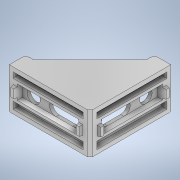
# Autodesk Inventor part: 3030 corner bracket 60x30
Saved by Autodesk Inventor 2022 (Build 260153000, 153)
## iProperties
Created: 2022-09-17
Part Number: 3030 corner bracket 60x30
Material: Genérico
Document SubType Name: Modeling
Designer: JK
Density: 1 g/cm^3
Appearance: Aluminio - Pulido
Author: JK
Autodesk Inventor part; units mm, degrees
note: some values were not read from the file. Chosen so that the rebuilt part matches the saved one: pattern direction of "Patrón circular2".
ref_plane "YZ Plane" through (0, 0, 0) normal (1, 0, 0) x (0, 1, 0)
ref_plane "XZ Plane" through (0, 0, 0) normal (0, 1, 0) x (-1, 0, 0)
ref_plane "XY Plane" through (0, 0, 0) normal (0, 0, 1) x (1, 0, 0)
sketch "Boceto1" plane through (0, 0, 0) normal (0, 1, 0) x (-1, 0, 0)
  line L0 (-29, 29) -> (29, 29)
  line L1 (29, 29) -> (29, -29)
  line L2 (29, -29) -> (-29, -29)
  line L3 (-29, -29) -> (-29, 29)
  line L4 (-29, 29) -> (29, -29) construction
  line L5 (29, 29) -> (-29, -29) construction
  line L6 (29, 23.4) -> (-23.4, 23.4)
  line L7 (-23.4, 23.4) -> (-23.4, -29)
  line L8 (-23.4, -29) -> (29, -29)
  line L9 (29, -29) -> (29, 23.4)
  point P0 (0, 0)
  dimension "d0" = 58
  dimension "d1" = 58
  dimension "d2" = 5.6
  dimension "d3" = 5.6
  constraints: 20 end point, 4 parallel, 2 horizontal, 2 midpoint, 2 perpendicular, 2 point on line
  measures "d0" distance of L1.end L2.end
  measures "d1" distance of L0.end L1.end
  measures "d2" distance between parallel lines of L6 L0
  measures "d3" distance between parallel lines of L3 L7
extrude "Extrusión1" add sketch "Boceto1" along normal mid plane 29.3 contours L0 L1 L6 L7 L2 L3
sketch "Boceto3" plane through (0, 14.65, 0) normal (0, 1, 0) x (1, 0, 0)
  line L0 (-29, -23.4) -> (-29, -29) projected
  line L1 (-29, -29) -> (-23.4, -29)
  line L2 (-23.4, -29) -> (-23.4, -17.2)
  line L3 (-23.4, -17.2) -> (-29, -17.2)
  line L4 (-29, -17.2) -> (-29, -29)
  line L5 (29, -29) -> (29, 29) projected
  line L6 (29, 29) -> (17.2, 29)
  line L7 (17.2, 29) -> (17.2, 23.4)
  line L8 (17.2, 23.4) -> (29, 23.4)
  line L9 (29, 23.4) -> (29, 29)
  line L10 (-23.4, -17.2) -> (17.2, 23.4)
  line L11 (29, -29) -> (29, 29) projected
  line L12 (29, 29) -> (23.4, 29) projected
  line L13 (23.4, 29) -> (23.4, -23.4) projected
  line L14 (23.4, -23.4) -> (-29, -23.4) projected
  line L15 (-29, -23.4) -> (-29, -29) projected
  line L16 (-29, -29) -> (29, -29) projected
  point P0 (0, 0)
  dimension "d7" = 11.8
  dimension "d8" = 11.8
  dimension "d9" = 5.6
  dimension "d10" = 5.6
  constraints: 18 end point, 4 parallel, 2 horizontal, 2 perpendicular
  measures "d7" distance between parallel lines of L16 L3
  measures "d8" distance between parallel lines of L9 L7
  measures "d9" distance of L2.end L3.end
  measures "d10" distance between parallel lines of L6 L8
extrude "Extrusión2" add sketch "Boceto3" against normal blind 3.25 contours L4 L3 L2 L14 | L2 L10 L8 L13 L14 | L7 L6 L13 L8
sketch "Boceto5" plane through (29, -14.65, -29) normal (1, 0, 0) x (0, 0, -1)
  line L0 (-53, 3) -> (-2.8, 3)
  line L1 (-2.8, 3) -> (-2.8, 8.3)
  line L2 (-2.8, 8.3) -> (-53, 8.3)
  line L3 (-53, 8.3) -> (-53, 3)
  line L4 (-53, 3) -> (-2.8, 8.3) construction
  line L5 (-2.8, 3) -> (-53, 8.3) construction
  line L6 (-53, 22.2) -> (-2.8, 22.2)
  line L7 (-2.8, 22.2) -> (-2.8, 26.2)
  line L8 (-2.8, 26.2) -> (-53, 26.2)
  line L9 (-53, 26.2) -> (-53, 22.2)
  line L10 (-53, 22.2) -> (-2.8, 26.2) construction
  line L11 (-2.8, 22.2) -> (-53, 26.2) construction
  line L12 (0, 0) -> (-58, 0) projected
  line L13 (-58, 29.3) -> (-58, 0) projected
  line L14 (-58, 29.3) -> (0, 29.3) projected
  line L15 (0, 0) -> (0, 29.3) projected
  line L16 (-53, 10.3) -> (-2.8, 10.3)
  line L17 (-2.8, 10.3) -> (-2.8, 20.2)
  line L18 (-2.8, 20.2) -> (-53, 20.2)
  line L19 (-53, 20.2) -> (-53, 10.3)
  line L20 (-53, 10.3) -> (-2.8, 20.2) construction
  line L21 (-2.8, 10.3) -> (-53, 20.2) construction
  point P0 (-29, 14.65)
  point P1 (-27.9, 5.65)
  point P2 (-27.9, 24.2)
  point P3 (-27.9, 15.25)
  dimension "d14" = 5.3
  dimension "d15" = 3
  dimension "d16" = 5
  dimension "d17" = 3.1
  dimension "d18" = 4
  dimension "d19" = 2.8
  dimension "d20" = 2
  dimension "d21" = 2
  constraints: 36 end point, 6 midpoint, 6 parallel, 3 collinear, 3 horizontal, 3 perpendicular, 1 point on line
  measures "d14" distance of L2.end L0.start
  measures "d15" distance between parallel lines of L12 L0
  measures "d16" distance between parallel lines of L13 L3
  measures "d17" distance between parallel lines of L14 L8
  measures "d18" distance of L8.end L6.start
  measures "d19" distance between parallel lines of L15 L1
  measures "d20" distance between parallel lines of L2 L16
  measures "d21" distance between parallel lines of L6 L18
extrude "Extrusión3" cut sketch "Boceto5" against normal blind 3.25 draft -8 contours L3 L2 L1 L0 | L9 L8 L7 L6 | L19 L18 L17 L16
sketch "Boceto6" plane through (-29, 14.65, 29) normal (0, 0, 1) x (1, 0, 0)
  line L0 (2.8, -26.3) -> (53, -26.3)
  line L1 (53, -26.3) -> (53, -21.3)
  line L2 (53, -21.3) -> (2.8, -21.3)
  line L3 (2.8, -21.3) -> (2.8, -26.3)
  line L4 (2.8, -26.3) -> (53, -21.3) construction
  line L5 (53, -26.3) -> (2.8, -21.3) construction
  line L6 (2.8, -7) -> (53, -7)
  line L7 (53, -7) -> (53, -3)
  line L8 (53, -3) -> (2.8, -3)
  line L9 (2.8, -3) -> (2.8, -7)
  line L10 (2.8, -7) -> (53, -3) construction
  line L11 (53, -7) -> (2.8, -3) construction
  line L12 (2.8, -19.3) -> (53, -19.3)
  line L13 (53, -19.3) -> (53, -9)
  line L14 (53, -9) -> (2.8, -9)
  line L15 (2.8, -9) -> (2.8, -19.3)
  line L16 (2.8, -19.3) -> (53, -9) construction
  line L17 (53, -19.3) -> (2.8, -9) construction
  line L18 (0, -29.3) -> (0, 0) projected
  line L19 (58, 0) -> (58, -29.3) projected
  line L20 (58, -3.1) -> (58, -7.1) projected
  line L21 (58, -7.1) -> (58, -3.1) projected
  line L22 (58, -9.1) -> (58, -19) projected
  line L23 (58, -19) -> (58, -9.1) projected
  line L24 (58, -21) -> (58, -26.3) projected
  line L25 (58, -26.3) -> (58, -21) projected
  line L26 (58, -29.3) -> (58, 0) projected
  line L27 (58, 0) -> (58, -29.3) projected
  line L28 (58, -29.3) -> (0, -29.3) projected
  line L29 (0, 0) -> (58, 0) projected
  point P0 (29, -14.65)
  point P1 (27.9, -23.8)
  point P2 (27.9, -5)
  point P3 (27.9, -14.15)
  dimension "d27" = 2.8
  dimension "d28" = 5
  dimension "d29" = 5
  dimension "d30" = 4
  dimension "d31" = 2
  dimension "d32" = 2
  dimension "d33" = 3
  dimension "d34" = 3
  constraints: 36 end point, 6 midpoint, 6 parallel, 4 collinear, 3 horizontal, 3 perpendicular
  measures "d27" distance between parallel lines of L18 L3
  measures "d28" distance between parallel lines of L19 L1
  measures "d29" distance between parallel lines of L0 L2
  measures "d30" distance between parallel lines of L8 L6
  measures "d31" distance between parallel lines of L12 L2
  measures "d32" distance between parallel lines of L6 L14
  measures "d33" distance between parallel lines of L28 L0
  measures "d34" distance between parallel lines of L29 L8
extrude "Extrusión4" cut sketch "Boceto6" against normal blind 3.25 draft -8 contours L3 L2 L1 L0 | L9 L8 L7 L6 | L15 L14 L13 L12
sketch "Boceto8" plane through (25.75, -14.65, -29) normal (1, 0, 0) x (0, 0, -1)
  circle A0 centre (-14.5932, 15.25) radius 4.4932
  circle A1 centre (-30.3797, 15.25) radius 4.4932
  circle A2 centre (-42.1932, 15.25) radius 4.4932
  line L0 (-30.3797, 19.7432) -> (-42.1932, 19.7432)
  line L1 (-42.1932, 19.7432) -> (-42.1932, 10.7568)
  line L2 (-42.1932, 10.7568) -> (-30.3797, 10.7568)
  line L3 (-30.3797, 10.7568) -> (-30.3797, 19.7432)
  line L4 (-3.2568, 19.7432) -> (-52.5432, 19.7432) projected
  line L5 (-52.5432, 19.7432) -> (-52.5432, 10.7568) projected
  line L6 (-52.5432, 10.7568) -> (-3.2568, 10.7568) projected
  line L7 (-3.2568, 10.7568) -> (-3.2568, 19.7432) projected
  line L8 (-3.2568, 19.7432) -> (-52.5432, 19.7432) projected
  line L9 (-52.5432, 10.7568) -> (-3.2568, 10.7568) projected
  line L10 (-10.1, 43.6813) -> (-10.1, -24.6831)
  line L11 (0, 0) -> (0, 29.3) projected
  line L12 (-25.8865, 40.14) -> (-25.8865, -28.2886)
  line L13 (-19.0865, 39.1194) -> (-19.0865, -26.6767)
  line L14 (-46.6865, 34.8598) -> (-46.6865, -29.8584)
  point P0 (-29, 14.65)
  point P1 (-42.1932, 19.7432)
  dimension "d45" = 10.1
  dimension "d46" = 6.8
  dimension "d47" = 20.8
  constraints: 16 end point, 5 tangent, 4 vertical, 3 horizontal, 3 parallel, 2 centre point, 2 collinear, 2 midpoint, 1 equal radius, 1 horizontal alignment, 1 perpendicular, 3 other
  measures "d45" distance between parallel lines of L11 L10
  measures "d46" distance between parallel lines of L13 L12
  measures "d47" distance between parallel lines of L14 L12
extrude "Extrusión6" cut sketch "Boceto8" against normal through all contours A0 | L3 A1 | A1 L2 A2 L0 | A1 L3 | L1 A2 | A2 L1
pattern_circular "Patrón circular2" count 2 over 90 about axis through (23.4, -14.65, 23.4) along (0, -1, 0) of "Extrusión6"
sketch "Boceto9" plane through (-29, 14.65, 25.75) normal (0, 0, 1) x (1, 0, 0)
  circle A0 centre (14.2762, -14.15) radius 4.6932
  circle A1 centre (30.38, -14.15) radius 4.6932
  circle A2 centre (42.194, -14.15) radius 4.6932
  line L0 (30.38, -18.8432) -> (42.194, -18.8432)
  line L1 (42.194, -18.8432) -> (42.194, -9.4568)
  line L2 (42.194, -9.4568) -> (30.38, -9.4568)
  line L3 (30.38, -9.4568) -> (30.38, -18.8432)
  line L4 (3.2568, -18.8432) -> (52.5432, -18.8432) projected
  line L5 (52.5432, -9.4568) -> (3.2568, -9.4568) projected
  line L6 (0, -29.3) -> (0, 0) projected
  point P0 (29, -14.65)
  dimension "d51" = 14.2762
  dimension "d52" = 30.38
  dimension "d53" = 11.814
  constraints: 8 end point, 5 tangent, 3 centre point, 2 collinear, 2 midpoint, 2 parallel, 1 coincident, 1 equal radius, 1 horizontal, 1 perpendicular
  measures "d51" distance from line of L6 A0.centre
  measures "d52" distance from line of L6 A1.centre
  measures "d53" distance of A1.centre A2.centre
extrude "Extrusión7" cut sketch "Boceto9" against normal through all contours A0 | L2 A2 L0 A1 | L3 A1 | A1 L3 | L1 A2 | A2 L1
fillet "Empalme1" radius 1 3 edges at (23.4, -1.625, 23.4) (23.4, 11.4, -2.8) (-2.8, 11.4, 23.4)
chamfer "Chaflán1" distance 2 angle 45 1 edges at (29, 0, 29)
fillet "Empalme2" radius 3 2 edges at (17.2, 13.025, -29) (-29, 13.025, 17.2)
fillet "Empalme3" radius 1 2 edges at (-23.4, 13.025, 17.2) (17.2, 13.025, -23.4)
fillet "Empalme4" radius 1 2 edges at (-29, -14.65, 26.2) (26.2, -14.65, -29)
sketch "Boceto11" plane through (29, -14.65, 27) normal (1, 0, 0) x (0, 0, -1)
  line L0 (3, 20.2) -> (53.2, 20.2) projected
  line L1 (53.2, 20.2) -> (50.2, 20.2)
  line L2 (50.2, 20.2) -> (50.2, 10.3)
  line L3 (50.2, 10.3) -> (53.2, 10.3)
  line L4 (53.2, 10.3) -> (53.2, 20.2)
  line L5 (3, 10.3) -> (6, 10.3)
  line L6 (6, 10.3) -> (6, 20.2)
  line L7 (6, 20.2) -> (3, 20.2)
  line L8 (3, 20.2) -> (3, 10.3)
  line L9 (53.2, 10.3) -> (3, 10.3) projected
  point P0 (27, 14.65)
  point P1 (6, 20.2)
  dimension "d63" = 3
  dimension "d64" = 3
  constraints: 16 end point, 4 parallel, 2 horizontal, 2 perpendicular, 2 point on line, 1 collinear
  measures "d63" distance between parallel lines of L6 L8
  measures "d64" distance between parallel lines of L4 L2
extrude "Extrusión8" add sketch "Boceto11" against normal up to surface (3.25 mm away) draft 8 contours L0 L6 L5 L8 | L0 L4 L3 L2
sketch "Boceto12" plane through (29, -14.65, 27) normal (1, 0, 0) x (0, 0, -1)
  line L0 (50.2, 20.2) -> (50.2, 10.3) projected
  line L1 (50.2, 11.3) -> (53, 11.3)
  line L2 (53, 11.3) -> (53, 18)
  line L3 (53, 18) -> (50.2, 18)
  line L4 (50.2, 18) -> (50.2, 11.3)
  line L5 (6, 10.3) -> (6, 20.2) projected
  line L6 (6, 11.3) -> (3.2, 11.3)
  line L7 (3.2, 11.3) -> (3.2, 18)
  line L8 (3.2, 18) -> (6, 18)
  line L9 (6, 18) -> (6, 11.3)
  line L10 (51.6, 11.3) -> (51.6, 0)
  line L11 (55, 0) -> (0, 0) projected
  line L12 (51.6, 18) -> (51.6, 29.3)
  line L13 (0, 29.3) -> (56, 29.3) projected
  point P0 (27, 14.65)
  point P1 (6, 18)
  dimension "d67" = 2.8
  dimension "d68" = 6.7
  constraints: 20 end point, 6 point on line, 4 parallel, 3 collinear, 2 horizontal, 2 midpoint, 2 perpendicular, 1 vertical
  measures "d67" distance of L1.start L1.end
  measures "d68" distance of L1.end L2.end
extrude "Extrusión9" add sketch "Boceto12" along normal blind 2.2 draft -8
sketch "Boceto13" plane through (-29, 14.65, 29) normal (0, 0, 1) x (1, 0, 0)
  line L0 (2.8, -9) -> (53, -9) projected
  line L1 (2.8, -9) -> (5.8, -9)
  line L2 (5.8, -9) -> (5.8, -19.3)
  line L3 (5.8, -19.3) -> (2.8, -19.3)
  line L4 (2.8, -19.3) -> (2.8, -9)
  line L5 (53, -9) -> (53, -19.3) projected
  line L6 (53, -19.3) -> (2.8, -19.3) projected
  line L7 (53, -9) -> (50, -9)
  line L8 (50, -9) -> (50, -19.3)
  line L9 (50, -19.3) -> (53, -19.3)
  line L10 (53, -19.3) -> (53, -9)
  point P0 (29, -14.65)
  point P1 (5.8, -9)
  dimension "d71" = 3
  dimension "d72" = 3
  constraints: 16 end point, 4 parallel, 2 horizontal, 2 perpendicular, 1 collinear, 1 point on line
  measures "d71" distance between parallel lines of L2 L4
  measures "d72" distance between parallel lines of L5 L8
extrude "Extrusión10" add sketch "Boceto13" against normal up to surface (3.25 mm away) draft 8 contours L0 L2 L3 L4 | L0 L5 L6 L8
sketch "Boceto14" plane through (-29, 14.65, 29) normal (0, 0, 1) x (1, 0, 0)
  line L0 (5.8, -19.3) -> (5.8, -9) projected
  line L1 (5.8, -10.9217) -> (3, -10.9217)
  line L2 (3, -10.9217) -> (3, -17.6217)
  line L3 (3, -17.6217) -> (5.8, -17.6217)
  line L4 (5.8, -17.6217) -> (5.8, -10.9217)
  line L5 (50, -9) -> (50, -19.3) projected
  line L6 (50, -10.9217) -> (52.8, -10.9217)
  line L7 (52.8, -10.9217) -> (52.8, -17.6217)
  line L8 (52.8, -17.6217) -> (50, -17.6217)
  line L9 (50, -17.6217) -> (50, -10.9217)
  line L10 (4.4, -10.9217) -> (4.4, 0.7566)
  line L11 (4.4, -17.6217) -> (4.4, -29.3)
  line L12 (56, -29.3) -> (1, -29.3) projected
  point P0 (29, -14.65)
  dimension "d75" = 6.7
  dimension "d76" = 2.8
  constraints: 20 end point, 4 parallel, 4 point on line, 3 collinear, 2 horizontal, 2 midpoint, 2 perpendicular, 2 vertical
  measures "d75" distance of L1.end L2.end
  measures "d76" distance of L1.start L1.end
extrude "Extrusión11" add sketch "Boceto14" along normal blind 2.2 draft -8
